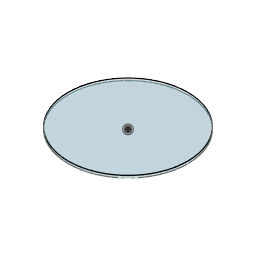
compass full assembly (Autodesk Fusion 360 archive; units mm, degrees)
design "top lid"
part number: 2026-06-30-18-08-59-397
Autodesk Fusion 360 part; units mm, degrees
sketch "Sketch1" plane through (0, 0, 0) normal (0, 1, 0) x (1, 0, 0)
  circle A0 centre (0, 0) radius 26
  dimension "d1" = 52
  constraint coincident A0.centre origin
  measures "d1" diameter of A0
extrude "Extrude1" add sketch "Sketch1" along normal blind 1
